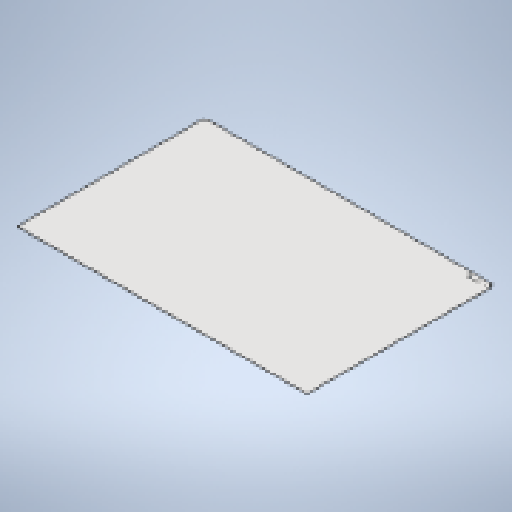
# Autodesk Inventor part: GnG frame 1.1 floor sheet 4
Saved by Autodesk Inventor 2025 (Build 290162010, 162A)
## iProperties
Created: 2025-10-28
Part Number: GnG frame 1.1 floor sheet 4
Material: Stainless Steel
Document SubType Name: Sheet Metal
Designer: admin
Mass: 453.26 g
Surface Area: 397.602 cm^2
Volume: 56.6575 cm^3
Density: 8 g/cm^3
Sheet Metal Rule: AISI304 3mm Die 32
Sheet Metal Width: 2300,000 mm
Sheet Metal Length: 1490,000 mm
Sheet Metal Area: 3427000,000 mm^2
Appearance: Default
Stock Number: 1.4
Flat Pattern Width: 230 cm
Flat Pattern Length: 149 cm
Flat Pattern Area: 34270 cm^2
Author: admin
Autodesk Inventor part; units mm, degrees
ref_plane "YZ Plane" through (0, 0, 0) normal (1, 0, 0) x (0, 1, 0)
ref_plane "XZ Plane" through (0, 0, 0) normal (0, 1, 0) x (-1, 0, 0)
ref_plane "XY Plane" through (0, 0, 0) normal (0, 0, 1) x (1, 0, 0)
sketch "Sketch1" plane through (0, 0, 0) normal (0, 0, 1) x (1, 0, 0)
  line L0 (0, 0) -> (-2300, 0)
  line L1 (-2300, 0) -> (-2300, -1490)
  line L2 (-2300, -1490) -> (0, -1490)
  line L3 (0, -1490) -> (0, 0)
  line L4 (0, 0) -> (-20, 0)
  line L5 (-20, 0) -> (-20, -20)
  line L6 (-20, -20) -> (0, -20)
  line L7 (0, -20) -> (0, 0)
  line L8 (0, -1490) -> (-20, -1490)
  line L9 (-20, -1490) -> (-20, -1470)
  line L10 (-20, -1470) -> (0, -1470)
  line L11 (0, -1470) -> (0, -1490)
  line L12 (-2300, 0) -> (-2280, 0)
  line L13 (-2280, 0) -> (-2280, -20)
  line L14 (-2280, -20) -> (-2300, -20)
  line L15 (-2300, -20) -> (-2300, 0)
  line L16 (-2300, -1490) -> (-2280, -1490)
  line L17 (-2280, -1490) -> (-2280, -1470)
  line L18 (-2280, -1470) -> (-2300, -1470)
  line L19 (-2300, -1470) -> (-2300, -1490)
  line L20 (-310, -1490) -> (-220, -1490)
  line L21 (-220, -1490) -> (-220, -1470)
  line L22 (-220, -1470) -> (-310, -1470)
  line L23 (-310, -1470) -> (-310, -1490)
  line L24 (-310, 0) -> (-220, 0)
  line L25 (-220, 0) -> (-220, -20)
  line L26 (-220, -20) -> (-310, -20)
  line L27 (-310, -20) -> (-310, 0)
  point P0 (0, -20)
  point P1 (-20, 0)
  point P2 (0, -1470)
  point P3 (-220, -1490)
  point P4 (-220, 0)
  point P5 (-2280, 0)
  dimension "d22" = 2300
  dimension "d23" = 1490
  dimension "d24" = 20
  dimension "d25" = 20
  dimension "d28" = 90
  dimension "d29" = 200
  measures "d22" distance of L2.end L1.end
  measures "d23" distance of L1.end L0.end
  measures "d24" distance of L6.end L5.end
  measures "d25" distance of L5.end L4.end
  measures "d28" distance of L25.end L26.end
  measures "d29" distance between parallel lines of L5 L25
extrude "Plate1" add sketch "Sketch1" along normal blind 3 contours L5 L6 L3 L10 L9 L2 L21 L22 L23 L17 L18 L1 L14 L13 L0 L27 L26 L25 | L25 L26 L27 L0 | L3 L2 L9 L10 | L2 L23 L22 L21 | L18 L17 L2 L1
sketch "Sketch5" plane through (0, 0, 3) normal (0, 0, 1) x (1, 0, 0)
  line L0 (105, 0) -> (110, 0)
  line L1 (114.9832, -0.8186) -> (119.9832, -0.8186)
  circle A0 centre (100, 0) radius 2.5
  line L2 (129.9832, -0.8186) -> (129.9832, -5)
  line L3 (134.9832, -0.8186) -> (136.3204, -4.2087)
  arc A1 (136.3204, -4.2087) -> (138.646, -4.2087) centre (137.4832, -3.75) ccw
  line L4 (134.9832, -0.8186) -> (139.9832, -0.8186)
  line L5 (129.9832, -0.8186) -> (134.9832, -0.8186) construction
  line L6 (138.646, -4.2087) -> (139.9832, -0.8186)
  line L7 (-1136.2996, -5.4093) -> (-1136.2996, -0.4093)
  line L8 (-1136.2996, -0.4093) -> (-1131.2996, -0.4093)
  line L9 (-1131.2996, -0.4093) -> (-1131.2996, -5.4093)
  line L10 (-1131.2996, -5.4093) -> (-1136.2996, -5.4093)
  line L11 (-1131.2996, -2.9093) -> (-1126.2996, -2.9093) construction
  line L12 (119.9832, -5) -> (114.9832, -5)
  line L13 (129.9832, -5) -> (124.9832, -5)
  line L14 (119.9832, -2.9093) -> (124.9832, -2.9093) construction
  line L15 (110, -2.5) -> (114.9832, -2.9093) construction
  line L16 (124.9832, -0.8186) -> (129.9832, -0.8186)
  line L17 (124.9832, -5) -> (124.9832, -0.8186)
  line L18 (119.9832, -0.8186) -> (119.9832, -5)
  line L19 (114.9832, -5) -> (114.9832, -0.8186)
  line L20 (110, 0) -> (110, -5)
  line L21 (105, -5) -> (105, 0)
  line L22 (110, -5) -> (105, -5)
  line L23 (-1126.2996, -5.4093) -> (-1126.2996, -0.4093)
  line L24 (-1121.2996, -5.4093) -> (-1126.2996, -5.4093)
  line L25 (-1126.2996, -0.4093) -> (-1121.2996, -0.4093)
  line L26 (-1121.2996, -0.4093) -> (-1121.2996, -5.4093)
  line L27 (-1121.2996, -2.9093) -> (-1116.2996, -2.9093) construction
  line L28 (-1116.2996, -5.4093) -> (-1116.2996, -0.4093)
  line L29 (-1116.2996, -0.4093) -> (-1111.2996, -0.4093)
  line L30 (-1111.2996, -0.4093) -> (-1111.2996, -5.4093)
  line L31 (-1111.2996, -5.4093) -> (-1116.2996, -5.4093)
  line L32 (-2280, 0) -> (0, 0) projected
  line L33 (-1101.2996, -5.8186) -> (-1106.2996, -5.8186)
  line L34 (-1106.2996, -5.8186) -> (-1106.2996, 0)
  line L35 (-1101.2996, 0) -> (-1101.2996, -5.8186)
  line L36 (-1106.2996, 0) -> (-1101.2996, 0)
  line L37 (-1106.2996, -2.9093) -> (-1111.2996, -2.9093)
  line L38 (-1154.9665, -0.6552) -> (-1153.6293, -4.0453)
  arc A2 (-1153.6293, -4.0453) -> (-1151.3037, -4.0453) centre (-1152.4665, -3.5866) ccw
  line L39 (-1154.9665, -0.6552) -> (-1149.9665, -0.6552)
  line L40 (-1151.3037, -4.0453) -> (-1149.9665, -0.6552)
  point P0 (137.4832, -0.8186)
  point P1 (-200, 0)
  point P2 (-1103.7996, 0)
  point P3 (-1101.2996, 0)
  point P4 (-1106.2996, 0)
  point P5 (-1152.4665, -0.6552)
  dimension "d30" = 5
  dimension "d31" = 5
  dimension "d32" = 1.25
  dimension "d33" = 5
  dimension "d34" = 5
  dimension "d35" = 5
  dimension "d36" = 5
  dimension "d37" = 5
  dimension "d38" = 300
  dimension "d41" = 1.25
  dimension "d42" = 5
  constraints: 80 end point, 14 parallel, 13 horizontal, 13 midpoint, 11 equal length, 7 perpendicular, 5 collinear, 5 tangent, 4 point on circle, 3 centre point, 3 point on line, 2 vertical alignment
  measures "d30" distance of L20.end L22.end
  measures "d31" distance of L22.end L0.start
  measures "d32" radius of A1
  measures "d33" distance of L5.end L4.end
  measures "d34" distance of L9.end L7.start
  measures "d35" distance of L7.start L7.end
  measures "d36" diameter of A0
  measures "d37" distance of A0.centre L0.start
  measures "d38" distance of point (-200, 0) A0.centre
  measures "d41" radius of A2
  measures "d42" distance of L38.start L39.end
cut "Cut1" [suppressed]
sketch "Sketch6" plane through (0, 0, 3) normal (0, 0, 1) x (1, 0, 0)
  circle A0 centre (-158.8151, -34.9821) radius 10
  point P0 (0, 0)
  dimension "d47" = 20
  constraints: 1 centre point
  measures "d47" diameter of A0
extrude "Cut2" cut sketch "Sketch6" against normal blind 3
sketch "Sketch7" plane through (0, 0, 0) normal (0, 0, -1) x (-1, 0, 0)
  circle A0 centre (158.8151, -34.9821) radius 10 projected
  line L0 (0, -1490) -> (0, -20) projected
  line L1 (2300, -1490) -> (0, -1490) projected
  line L2 (2300, -20) -> (2300, -1490) projected
  line L3 (2280, -20) -> (2300, -20) projected
  line L4 (2280, 0) -> (2280, -20) projected
  line L5 (20, 0) -> (2280, 0) projected
  line L6 (20, -20) -> (20, 0) projected
  line L7 (0, -20) -> (20, -20) projected
  line L8 (18.9195, -35.9471) -> (103.9529, -35.9471) construction
  line L9 (103.9529, -35.9471) -> (103.9529, -51.8936) construction
  line L10 (103.9529, -51.8936) -> (18.9195, -51.8936) construction
  line L11 (18.9195, -51.8936) -> (18.9195, -35.9471) construction
  point P0 (0, 0)
  constraints: 2 other
mark "Mark2"
equation "\"d24\" = d25"
equation "\"d32\" = 0.25 * d30"
equation "\"d41\" = 0.25 * d43"
equation "\"d39\" = Thickness"
equation "\"d48\" = Thickness"
equation "\"d2\" = Thickness"
equation "\"BendReliefWidth\" = Thickness"
equation "\"BendReliefDepth\" = 0.5 * Thickness"
equation "\"CornerReliefSize\" = 4 * Thickness"
equation "\"MinimumRemnant\" = 2 * Thickness"
equation "\"TransitionRadius\" = BendRadius"
equation "\"JacobiRadiusSize\" = BendRadius"
equation "\"GapSize\" = Thickness"
equation "\"d43\" = 5"
equation "\"Thickness\" = 3"
equation "\"BendRadius\" = 5"
body "Solid1"
